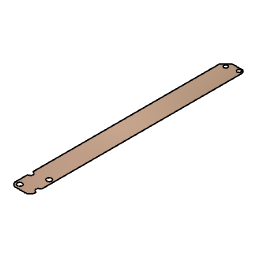
copper braid specimen cooling v4 (Autodesk Fusion 360 design; units mm, degrees)
Autodesk Fusion 360 part; units mm, degrees
note: some values were not read from the file. Set by a fixed rule: the direction of a hole.
sketch "Sketch1" plane through (0, 0, 0) normal (0, 1, 0) x (1, 0, 0)
  line L0 (0, 0) -> (18, 0)
  line L1 (18, 0) -> (18, -200)
  line L2 (18, -200) -> (0, -200)
  line L3 (0, -200) -> (0, 0)
  circle A0 centre (9, -187) radius 10
  line L4 (9, -187) -> (19, -187) construction
  line L5 (9, -187) -> (14, -178.3397) construction
  line L6 (9, -200) -> (9, -187) construction
  line L7 (5, -5) -> (14.6593, -2.4118) construction
  point P0 (5, -5)
  point P1 (14.6593, -2.4118)
  point P2 (14, -178.3397)
  point P3 (0.3397, -182)
  point P4 (4, -195.6603)
  point P5 (17.6603, -192)
  dimension "d1" = 18
  dimension "d2" = 200
  dimension "d3" = 10
  dimension "d4" = 5
  dimension "d5" = 5
  dimension "d12" = 20
  dimension "d13" = 60
  dimension "d14" = 13
  dimension "d19" = 360
  dimension "d20" = 15
  constraint horizontal L0
  constraint vertical L1
  constraint horizontal L2
  constraint vertical L3
  constraint coincident L0.start L3.end
  constraint coincident A0.centre L4.start
  constraint perpendicular L1 L4
  constraint coincident A0 P2
  constraint coincident A0 L4.end
  constraint coincident P2 L5.end
  constraint midpoint L2 L6.start
  constraint vertical L6
  constraint coincident P0 L7.start
  constraint coincident P1 L7.end
  measures "d1" distance of L0.start L0.end
  measures "d2" distance of L0.end L1.end
  measures "d3" distance of P0 P1
  measures "d4" distance of L3 P0
  measures "d5" distance of L0 P0
  measures "d12" diameter of A0
  measures "d13" angle of L4 L5
  measures "d14" distance of L6.start A0.centre
  measures "d20" angle of L0 L7
extrude "Extrude1" add sketch "Sketch1" along normal blind 0.05 contours L0 L1 L3 A0 | L1 L3 A0 | L1 L2 L3 A0
hole "Hole1" at (5, 0, 5) at (14.6593, 0, 2.4118) direction (0, 1, 0) diameter 3.5 end through all
chamfer "Chamfer1" distance 3 angle 45 2 edges at (18, 0.025, 200) (0, 0.025, 200)
hole "Hole2" at (14, 0, 178.3397) at (0.3397, 0, 182) at (4, 0, 195.6603) at (17.6603, 0, 192) direction (0, 1, 0) diameter 4.5 depth 0.05 tip angle 118
chamfer "Chamfer2" distance 2 angle 45 1 edges at (18, 0.025, 0)
chamfer "Chamfer3" distance 6 angle 45 1 edges at (0, 0.025, 0)
